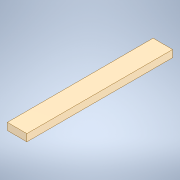
# Autodesk Inventor part: Балка РБАСУ
Saved by Autodesk Inventor 2022 (Build 260153000, 153)
## iProperties
Created: 2022-05-03
Part Number: Балка РБАСУ
Material: Пластик АБС
Document SubType Name: Modeling
Designer: Кочетов.А.И.
Density: 1.06 g/cm^3
Appearance: Гладкий — серовато-белый
Author: Кочетов.А.И.
Autodesk Inventor part; units mm, degrees
ref_plane "YZ Plane" through (0, 0, 0) normal (1, 0, 0) x (0, 1, 0)
ref_plane "XZ Plane" through (0, 0, 0) normal (0, 1, 0) x (-1, 0, 0)
ref_plane "XY Plane" through (0, 0, 0) normal (0, 0, 1) x (1, 0, 0)
sketch "Эскиз1" plane through (0, 0, 0) normal (0, 1, 0) x (-1, 0, 0)
  line L0 (-2.75, 20.5) -> (2.75, 20.5)
  line L1 (2.75, 20.5) -> (2.75, -20.5)
  line L2 (2.75, -20.5) -> (-2.75, -20.5)
  line L3 (-2.75, -20.5) -> (-2.75, 20.5)
  line L4 (-2.75, 20.5) -> (2.75, -20.5) construction
  line L5 (2.75, 20.5) -> (-2.75, -20.5) construction
  point P0 (0, 0)
  dimension "d0" = 5.5
  dimension "d1" = 41
  constraints: 12 end point, 2 midpoint, 2 parallel, 1 horizontal, 1 perpendicular
  measures "d0" distance between parallel lines of L3 L1
  measures "d1" distance between parallel lines of L0 L2
extrude "Выдавливание1" add sketch "Эскиз1" along normal blind 2
